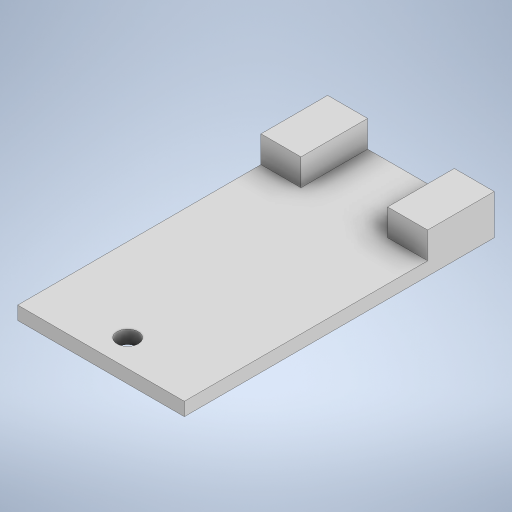
# Autodesk Inventor part: mlx_mount_3mm
Saved by Autodesk Inventor 2023 (Build 270158000, 158)
## iProperties
Created: 2023-10-27
Part Number: mlx_mount_3mm
Material: Generic
Document SubType Name: Modeling
Designer: mark
Density: 1 g/cm^3
Appearance: Default
Author: mark
Autodesk Inventor part; units mm, degrees
ref_plane "YZ Plane" through (0, 0, 0) normal (1, 0, 0) x (0, 1, 0)
ref_plane "XZ Plane" through (0, 0, 0) normal (0, 1, 0) x (-1, 0, 0)
ref_plane "XY Plane" through (0, 0, 0) normal (0, 0, 1) x (1, 0, 0)
sketch "Sketch1" plane through (0, 0, 0) normal (0, 1, 0) x (-1, 0, 0)
  line L0 (0, 0) -> (-25, 0)
  line L1 (-25, 0) -> (-25, -46.5)
  line L2 (-25, -46.5) -> (0, -46.5)
  line L3 (0, -46.5) -> (0, 0)
  dimension "d0" = 25
  dimension "d1" = 46.5
  constraints: 8 end point, 2 parallel, 1 horizontal, 1 perpendicular
  measures "d0" distance of L2.end L1.end
  measures "d1" distance of L1.end L0.end
extrude "Extrusion1" add sketch "Sketch1" along normal blind 2
sketch "Sketch2" plane through (0, 2, 0) normal (0, 1, 0) x (1, 0, 0)
  line L0 (25, 46.5) -> (0, 46.5) projected
  line L1 (0, 46.5) -> (6, 46.5)
  line L2 (6, 46.5) -> (6, 36.5)
  line L3 (6, 36.5) -> (0, 36.5)
  line L4 (0, 36.5) -> (0, 46.5)
  line L5 (25, 46.5) -> (19, 46.5)
  line L6 (19, 46.5) -> (19, 36.5)
  line L7 (19, 36.5) -> (25, 36.5)
  line L8 (25, 36.5) -> (25, 46.5)
  point P0 (0, 0)
  dimension "d4" = 6
  dimension "d5" = 10
  dimension "d6" = 6
  constraints: 16 end point, 4 parallel, 2 horizontal, 2 perpendicular, 1 point on line
  measures "d4" distance of L2.end L3.end
  measures "d5" distance of L1.end L2.end
  measures "d6" distance of L7.end L6.end
extrude "Extrusion2" add sketch "Sketch2" along normal blind 4
sketch "Sketch4" plane through (0, 2, 0) normal (0, 1, 0) x (1, 0, 0)
  line L0 (0, 0) -> (25, 0) projected
  line L1 (25, 0) -> (25, 36.5) projected
  point P0 (12.5, 4)
  dimension "d18" = 4
  dimension "d19" = 12.5
  measures "d18" distance from line of L0 point (12.5, 4)
  measures "d19" distance from line of L1 point (12.5, 4)
hole "Hole2" at (12.5, 2, -4) direction (0, -1, 0) diameter 3.2 end through all
body "Solid1"
